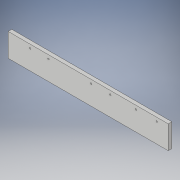
# Autodesk Inventor part: Kermit bumper (midlde 3)
Saved by Autodesk Inventor 2018.2 (Build 222227000, 227)
## iProperties
Created: 2018-02-15
Part Number: Kermit bumper (midlde 3)
Material: Generic
Document SubType Name: Modeling
Designer: kalra.rohan
Density: 1 g/cm^3
Appearance: Default
Author: kalra.rohan
Autodesk Inventor part; units mm, degrees
ref_plane "YZ Plane" through (0, 0, 0) normal (1, 0, 0) x (0, 1, 0)
ref_plane "XZ Plane" through (0, 0, 0) normal (0, 1, 0) x (-1, 0, 0)
ref_plane "XY Plane" through (0, 0, 0) normal (0, 0, 1) x (1, 0, 0)
sketch "Sketch1" plane through (0, 0, 0) normal (0, 0, 1) x (1, 0, 0)
  line L0 (0, 0) -> (831.85, 0)
  line L1 (831.85, 0) -> (831.85, -120.65)
  line L2 (831.85, -120.65) -> (0, -120.65)
  line L3 (0, -120.65) -> (0, 0)
  circle A0 centre (114.3, -19.05) radius 3.8671
  circle A1 centre (209.55, -19.05) radius 3.8671
  circle A2 centre (431.8, -19.05) radius 3.8735
  circle A3 centre (530.86, -19.05) radius 3.8735
  circle A4 centre (664.21, -19.05) radius 3.8735
  circle A5 centre (772.16, -19.05) radius 3.8671
  dimension "d0" = 831.85
  dimension "d1" = 120.65
  dimension "d2" = 101.6
  dimension "d3" = 7.7343
  dimension "d4" = 114.3
  dimension "d5" = 7.7343
  dimension "d6" = 95.25
  dimension "d7" = 7.747
  dimension "d9" = 101.6
  dimension "d10" = 222.25
  dimension "d11" = 7.747
  dimension "d12" = 101.6
  dimension "d13" = 99.06
  dimension "d14" = 7.747
  dimension "d15" = 101.6
  dimension "d16" = 133.35
  dimension "d17" = 7.7343
  dimension "d18" = 107.95
  constraints: 8 end point, 6 centre point, 2 parallel, 1 horizontal, 1 perpendicular
  measures "d0" distance between parallel lines of L1 L3
  measures "d1" distance between parallel lines of L0 L2
  measures "d2" distance from line of A0.centre L2
  measures "d3" diameter of A0
  measures "d4" distance from line of A0.centre L3
  measures "d5" diameter of A1
  measures "d6" distance of A1.centre A0.centre
  measures "d7" diameter of A2
  measures "d9" distance from line of A2.centre L2
  measures "d10" distance of A2.centre A1.centre
  measures "d11" diameter of A3
  measures "d12" distance from line of A3.centre L2
  measures "d13" distance of A3.centre A2.centre
  measures "d14" diameter of A4
  measures "d15" distance from line of L2 A4.centre
  measures "d16" distance of A4.centre A3.centre
  measures "d17" diameter of A5
  measures "d18" distance of A5.centre A4.centre
extrude "Extrusion1" add sketch "Sketch1" along normal blind 19.05
body "Solid1"
